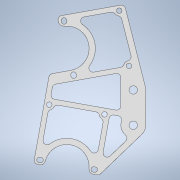
# Autodesk Inventor part: Knee_side_frame
Saved by Autodesk Inventor 2020 (Build 240168000, 168)
## iProperties
Created: 2021-09-05
Part Number: Knee_side_frame
Material: アルミニウム 2014-T4
Document SubType Name: Modeling
Designer: Masato Kubotera
Density: 2.8 g/cm^3
Appearance: 滑らか - 淡い灰色
Mass: 7.94371 g
Surface Area: 42.7962 cm^2
Volume: 2.83704 cm^3
Description: A2017 T2
Author: Masato Kubotera
Autodesk Inventor part; units mm, degrees
ref_plane "YZ Plane" through (0, 0, 0) normal (1, 0, 0) x (0, 1, 0)
ref_plane "XZ Plane" through (0, 0, 0) normal (0, 1, 0) x (-1, 0, 0)
ref_plane "XY Plane" through (0, 0, 0) normal (0, 0, 1) x (1, 0, 0)
sketch "スケッチ1" plane through (0, 0, 0) normal (0, 0, 1) x (1, 0, 0)
  line L0 (-14.5961, 13.6731) -> (27.7507, 21.14) construction
  line L1 (27.7507, 21.14) -> (33.3074, -10.3738) construction
  line L2 (33.3074, -10.3738) -> (-9.0393, -17.8407) construction
  line L3 (-9.0393, -17.8407) -> (-14.5961, 13.6731) construction
  line L4 (-14.5961, 13.6731) -> (33.3074, -10.3738) construction
  line L5 (27.7507, 21.14) -> (-9.0393, -17.8407) construction
  line L6 (-11.8177, -2.0838) -> (30.529, 5.3831) construction
  line L7 (25.2304, 18.1571) -> (-1.3594, 13.4686) construction
  line L8 (-1.3594, 13.4686) -> (3.3291, -13.1213) construction
  line L9 (3.3291, -13.1213) -> (29.9189, -8.4328) construction
  line L10 (29.9189, -8.4328) -> (25.2304, 18.1571) construction
  line L11 (25.2304, 18.1571) -> (3.3291, -13.1213) construction
  line L12 (-1.3594, 13.4686) -> (29.9189, -8.4328) construction
  circle A0 centre (0, 0) radius 10.5 construction
  line L13 (11.9355, 15.8128) -> (16.624, -10.777) construction
  circle A1 centre (25.2304, 18.1571) radius 1.35
  circle A2 centre (29.9189, -8.4328) radius 1.35
  arc A3 (-4.1041, 12.9846) -> (-1.0796, 10.6957) centre (-1.3594, 13.4686) ccw
  line L14 (-4.1041, 12.9846) -> (-4.5382, 15.4466)
  circle A4 centre (32, -20) radius 2.05
  circle A5 centre (32, -20) radius 6 construction
  circle A6 centre (32, -20) radius 4.6 construction
  line L15 (-4.5382, 15.4466) -> (27.7507, 21.14)
  line L16 (27.7507, 21.14) -> (37.8157, -18.5242)
  arc A7 (38, -20) -> (37.8157, -18.5242) centre (32, -20) ccw
  circle A8 centre (0, -57) radius 10.5 construction
  line L17 (0.2262, 13.7481) -> (22.7683, 17.7229)
  arc A9 (4.9147, -12.8417) -> (0.2262, 13.7481) centre (0, 0) ccw
  line L18 (4.9147, -12.8417) -> (27.4568, -8.8669)
  line L19 (26.0149, 15.7833) -> (31.7198, -6.6988)
  arc A10 (22.7683, 17.7229) -> (26.0149, 15.7833) centre (25.2304, 18.1571) ccw
  arc A11 (31.7198, -6.6988) -> (27.4568, -8.8669) centre (29.9189, -8.4328) ccw
  arc A12 (-0.03, 13.703) -> (-2.6889, 13.2341) centre (-1.3594, 13.4686) ccw
  arc A13 (-2.6021, 12.7417) -> (0.0569, 13.2106) centre (-1.2726, 12.9761) ccw
  line L20 (-2.6889, 13.2341) -> (-2.6021, 12.7417)
  line L21 (0.0569, 13.2106) -> (-0.03, 13.703)
  arc A14 (1.9996, -13.3557) -> (4.6585, -12.8868) centre (3.3291, -13.1213) ccw
  arc A15 (4.5717, -12.3944) -> (1.9127, -12.8633) centre (3.2422, -12.6289) ccw
  line L22 (1.9996, -13.3557) -> (1.9127, -12.8633)
  line L23 (4.5717, -12.3944) -> (4.6585, -12.8868)
  line L24 (-17.8407, -66.0393) -> (-10.3738, -23.6926) construction
  line L25 (-10.3738, -23.6926) -> (21.14, -29.2493) construction
  line L26 (21.14, -29.2493) -> (13.6731, -71.5961) construction
  line L27 (13.6731, -71.5961) -> (-17.8407, -66.0393) construction
  line L28 (-17.8407, -66.0393) -> (21.14, -29.2493) construction
  line L29 (-10.3738, -23.6926) -> (13.6731, -71.5961) construction
  line L30 (-2.0838, -68.8177) -> (5.3831, -26.471) construction
  line L31 (13.4686, -58.3594) -> (18.1571, -31.7696) construction
  line L32 (18.1571, -31.7696) -> (-8.4328, -27.0811) construction
  line L33 (-8.4328, -27.0811) -> (-13.1213, -53.6709) construction
  line L34 (-13.1213, -53.6709) -> (13.4686, -58.3594) construction
  line L35 (13.4686, -58.3594) -> (-8.4328, -27.0811) construction
  line L36 (18.1571, -31.7696) -> (-13.1213, -53.6709) construction
  circle A16 centre (-8.4328, -27.0811) radius 1.35
  arc A17 (-12.8868, -52.3415) -> (-13.3557, -55.0004) centre (-13.1213, -53.6709) ccw
  line L37 (-12.8868, -52.3415) -> (-12.3944, -52.4283)
  line L38 (-12.8633, -55.0873) -> (-13.3557, -55.0004)
  arc A18 (-12.8633, -55.0873) -> (-12.3944, -52.4283) centre (-12.6289, -53.7578) ccw
  line L39 (0, -57) -> (0, 0) construction
  line L40 (18.1571, -31.7696) -> (13.4686, -58.3594) construction
  circle A19 centre (18.1571, -31.7696) radius 1.35
  arc A20 (13.2341, -59.6889) -> (13.703, -57.03) centre (13.4686, -58.3594) ccw
  line L41 (13.703, -57.03) -> (13.2106, -56.9431)
  line L42 (12.7417, -59.6021) -> (13.2341, -59.6889)
  arc A21 (13.2106, -56.9431) -> (12.7417, -59.6021) centre (12.9761, -58.2726) ccw
  circle A22 centre (32, -37) radius 2.05
  circle A23 centre (32, -37) radius 6 construction
  line L43 (32, -20) -> (32, -37) construction
  arc A24 (1.8667, -10.5867) -> (-1.0796, 10.6957) centre (0, 0) ccw
  arc A25 (10.6987, -58.0493) -> (-10.4123, -54.3268) centre (0, -57) ccw
  arc A26 (11.5186, -49.491) -> (-8.2557, -46.0043) centre (0, -57) ccw
  line L44 (-15.9807, -55.4905) -> (-13.0262, -56.0114)
  arc A27 (-13.0262, -56.0114) -> (-10.4123, -54.3268) centre (-12.6289, -53.7578) ccw
  arc A28 (10.6987, -58.0493) -> (12.5788, -60.5263) centre (12.9761, -58.2726) ccw
  line L45 (15.5332, -61.0472) -> (36.1466, -41.3365)
  line L46 (38, -37) -> (38, -20)
  arc A29 (36.1466, -41.3365) -> (38, -37) centre (32, -37) ccw
  line L47 (16.4135, -56.0547) -> (30.3178, -42.7593)
  arc A30 (-8.8669, -29.5432) -> (-5.9337, -27.0141) centre (-8.4328, -27.0811) ccw
  line L48 (-11.4262, -44.0576) -> (-8.8669, -29.5432)
  line L49 (-5.9337, -27.0141) -> (15.8316, -30.8519)
  arc A31 (15.8316, -30.8519) -> (17.7229, -34.2317) centre (18.1571, -31.7696) ccw
  line L50 (15.1636, -48.7461) -> (17.7229, -34.2317)
  line L51 (20.6191, -32.2038) -> (16.4135, -56.0547)
  circle A32 centre (18.1571, -31.7696) radius 2.4 construction
  arc A33 (-9.98, -12.506) -> (2.7784, -15.7569) centre (0, 0) ccw construction
  line L52 (-8.7981, -23.9704) -> (-7.3221, -15.5996) construction
  line L53 (-7.3221, -15.5996) -> (21.0403, -20.6006) construction
  line L54 (19.5643, -28.9715) -> (21.0403, -20.6006) construction
  line L55 (12.5788, -60.5263) -> (15.5332, -61.0472)
  line L56 (-15.9807, -55.4905) -> (-8.3815, -12.3937)
  line L57 (-8.3815, -12.3937) -> (1.8667, -10.5867)
  arc A34 (20.6191, -32.2038) -> (20.6562, -31.7026) centre (18.1571, -31.7696) ccw
  line L58 (20.6562, -31.7026) -> (27.5951, -32.9261)
  arc A35 (27.5951, -32.9261) -> (30.3178, -42.7593) centre (32, -37) ccw
  line L59 (-6.7317, -17.4338) -> (-7.9118, -24.1267)
  line L60 (-7.9118, -24.1267) -> (26, -30.1063)
  line L61 (26, -30.1063) -> (26, -11.6623)
  line L62 (-6.7317, -17.4338) -> (26, -11.6623)
  arc A36 (-11.4262, -44.0576) -> (-8.2557, -46.0043) centre (-9.4566, -44.4049) ccw
  arc A37 (11.5186, -49.491) -> (15.1636, -48.7461) centre (13.194, -48.3988) ccw
  point P0 (9.3557, 1.6497)
  point P1 (14.2797, 2.5179)
  point P2 (1.6497, -47.6443)
  point P3 (2.5179, -42.7203)
  point P4 (2.5179, -42.7203)
  point P5 (-12.8417, -52.0853)
  point P6 (13.7481, -56.7738)
  point P7 (31.7198, -6.6988)
  point P8 (-13.0711, -52.3219)
  point P9 (-12.9341, -52.334)
  point P10 (13.7499, -57.0391)
  point P11 (13.8829, -57.0746)
  dimension "d21" = 43
  dimension "d22" = 32
  dimension "d23" = 27
  dimension "d24" = 27
  dimension "d27" = 21
  dimension "d28" = 9.5
  dimension "d31" = 4.1
  dimension "d34" = 12
  dimension "d39" = 8.5
  dimension "d40" = 9.2
  dimension "d41" = 32
  dimension "d46" = 20
  dimension "d56" = 2.5
  dimension "d57" = 2.5
  dimension "d62" = 3
  dimension "d63" = 2.5
  dimension "d67" = 2.7
  dimension "d68" = 1.35
  dimension "d70" = 0.5
  dimension "d72" = 43
  dimension "d73" = 32
  dimension "d77" = 9.5
  dimension "d78" = 20
  dimension "d80" = 27
  dimension "d81" = 27
  dimension "d82" = 8.5
  dimension "d83" = 2.7
  dimension "d86" = 0.5
  dimension "d87" = 1.35
  dimension "d88" = 57
  dimension "d89" = 80
  dimension "d90" = 21
  dimension "d91" = 100
  dimension "d92" = 4.1
  dimension "d93" = 12
  dimension "d94" = 17
  dimension "d95" = 3
  dimension "d96" = 0.25
  dimension "d97" = 0.25
  dimension "d98" = 3
  dimension "d99" = 0
  dimension "d101" = 2.5
  dimension "d102" = 3
  dimension "d107" = 2.5
  dimension "d109" = 2.5
  dimension "d111" = 4.8
  dimension "d112" = 8.5
  dimension "d113" = 28.8
  dimension "d114" = 2.5
  dimension "d115" = 2.5
  dimension "d116" = 2
  dimension "d117" = 2
  dimension "d118" = 2.5
  dimension "d119" = 2.5
  dimension "d120" = 2.5
  constraints: 126 end point, 61 point on circle, 38 centre point, 24 coincident, 22 parallel, 22 symmetric about line, 22 tangent, 16 point on line, 15 midpoint, 11 perpendicular, 2 collinear, 2 vertical, 1 concentric, 8 other
  measures "d21" distance of L1.end L2.end
  measures "d22" distance of L0.end L1.end
  measures "d23" distance of L9.end L8.end
  measures "d24" distance of L8.end L7.end
  measures "d27" diameter of A0
  measures "d28" distance of point (9.356, 1.65) A0.centre
  measures "d31" diameter of A4
  measures "d34" diameter of A5
  measures "d39" distance from line of L8 point (9.356, 1.65)
  measures "d40" diameter of A6
  measures "d41" horizontal distance of A4.centre A0.centre
  measures "d46" vertical distance of L43.start A0.centre
  measures "d56" radius of A10
  measures "d57" distance from line of L17.end L15
  measures "d62" distance between parallel lines of L16 L19
  measures "d63" radius of A11
  measures "d67" diameter of A1
  measures "d68" radius of A12
  measures "d70" distance of L21.start L21.end
  measures "d72" distance of L25.end L26.end
  measures "d73" distance of L24.end L25.end
  measures "d77" distance of L39.start point (1.65, -47.644)
  measures "d78" angle of L25 L2
  measures "d80" distance of L31.start L31.end
  measures "d81" distance of L31.end L32.end
  measures "d82" distance from line of L34 point (1.65, -47.644)
  measures "d83" diameter of A16
  measures "d86" distance of L33.end A18.centre
  measures "d87" radius of A17
  measures "d88" distance of L39.start A0.centre
  measures "d89" angle of L39 L2
  measures "d90" diameter of A8
  measures "d91" angle of L25 L39
  measures "d92" diameter of A22
  measures "d93" diameter of A23
  measures "d94" distance of L43.start L43.end
  measures "d95" radial gap between concentric circles of A24 A9
  measures "d96" radial gap between concentric circles of A0 A24
  measures "d97" radial gap between concentric circles of A8 A25
  measures "d98" radial gap between concentric circles of A25 A26
  measures "d99" distance between parallel lines of L9 L18
  measures "d101" radius of A30
  measures "d102" distance between parallel lines of L45 L47
  measures "d107" distance between parallel lines of L49 L25
  measures "d109" distance between parallel lines of L50 L51
  measures "d111" diameter of A32
  measures "d112" distance of L52.start L52.end
  measures "d113" distance of L52.end L53.end
  measures "d114" distance between parallel lines of L56 L48
  measures "d115" radius of A34
  measures "d116" radius of A36
  measures "d117" radius of A37
  measures "d118" distance between parallel lines of L49 L60
  measures "d119" distance between parallel lines of L56 L59
  measures "d120" distance between parallel lines of L62 L18
extrude "押し出し1" add sketch "スケッチ1" along normal blind 2
fillet "フィレット1" radius 2 6 edges at (-4.5382, 15.4466, 1) (27.7507, 21.14, 1) (15.5332, -61.0472, 1) (-15.9807, -55.4905, 1) (1.8667, -10.5867, 1) (-8.3815, -12.3937, 1)
fillet "フィレット2" radius 2 19 edges at (0.2262, 13.7481, 1) (4.9147, -12.8417, 1) (27.4568, -8.8669, 1) (22.7683, 17.7229, 1) (26.0149, 15.7833, 1) (-8.8669, -29.5432, 1) (16.4135, -56.0547, 1) (-5.9337, -27.0141, 1) (17.7229, -34.2317, 1) (15.8316, -30.8519, 1) (-7.9118, -24.1267, 1) (-6.7317, -17.4338, 1) (27.5951, -32.9261, 1) (20.6562, -31.7026, 1) (20.6191, -32.2038, 1) (30.3178, -42.7593, 1) (26, -30.1063, 1) (26, -11.6623, 1) (31.7198, -6.6988, 1)
